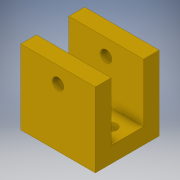
# Autodesk Inventor part: BracketForEndOfArm
Saved by Autodesk Inventor 2017 SP1 (Build 210196100, 196)
## iProperties
Created: 2016-06-07
Part Number: BracketForEndOfArm
Material: Generic
Document SubType Name: Modeling
Designer: steele
Density: 1 g/cm^3
Appearance: Gold
Author: steele
Autodesk Inventor part; units mm, degrees
ref_plane "YZ Plane" through (0, 0, 0) normal (1, 0, 0) x (0, 1, 0)
ref_plane "XZ Plane" through (0, 0, 0) normal (0, 1, 0) x (-1, 0, 0)
ref_plane "XY Plane" through (0, 0, 0) normal (0, 0, 1) x (1, 0, 0)
sketch "Sketch2" plane through (0, 0, 0) normal (1, 0, 0) x (0, 1, 0)
  line L0 (0, 0) -> (0, -19.05)
  line L1 (0, -19.05) -> (44.45, -19.05)
  line L2 (44.45, -19.05) -> (44.45, -9.652)
  line L3 (44.45, -9.652) -> (9.525, -9.652)
  line L4 (9.525, -9.652) -> (9.525, 0)
  line L5 (9.525, 0) -> (0, 0) construction
  line L6 (0, 0) -> (0, 19.05)
  line L7 (0, 19.05) -> (44.45, 19.05)
  line L8 (44.45, 19.05) -> (44.45, 9.652)
  line L9 (44.45, 9.652) -> (9.525, 9.652)
  line L10 (9.525, 9.652) -> (9.525, 0)
  dimension "d5" = 44.45
  dimension "d7" = 9.398
  dimension "d8" = 9.525
  dimension "d42" = 9.652
  constraints: 22 end point, 4 symmetric about line, 3 perpendicular, 2 vertical, 1 horizontal
  measures "d5" distance of L0.end L1.end
  measures "d7" distance between parallel lines of L1 L3
  measures "d8" distance between parallel lines of L0 L4
  measures "d42" distance from line of L0.start L3
extrude "Extrusion2" add sketch "Sketch2" along normal mid plane 44.45
sketch "Sketch3" plane through (-22.225, 0, 19.05) normal (0, 0, 1) x (1, 0, 0)
  line L0 (0, 44.45) -> (44.45, 44.45) projected
  line L1 (22.225, 44.45) -> (22.225, 0) construction
  point P0 (22.225, 34.925)
  dimension "d19" = 9.525
  constraints: 2 end point, 1 midpoint, 1 point on line, 1 vertical
  measures "d19" distance from line of point (22.225, 34.925) L0
hole "Hole2" at (0, 34.925, 19.05) direction (0, 0, -1) diameter 6.7564 end through all clearance for "Flat Head Machine Screw (82)" size "1/4" standard "Ansi Unified Screw Threads"
sketch "Sketch4" plane through (-22.225, 0, -19.05) normal (0, -1, 0) x (1, 0, 0)
  line L0 (44.45, 9.398) -> (44.45, 28.702) construction
  line L1 (44.45, 19.05) -> (0, 19.05) construction
  line L2 (0, 28.702) -> (0, 9.398) construction
  line L3 (44.45, 38.1) -> (44.45, 0) construction
  line L4 (19.05, 19.05) -> (-25.4, 19.05) construction
  point P0 (22.225, 19.05)
  point P1 (34.925, 19.05)
  point P2 (9.525, 19.05)
  dimension "d27" = 9.525
  dimension "d30" = 25.4
  constraints: 4 end point, 2 midpoint, 2 point on line, 1 collinear, 1 horizontal, 3 other
  measures "d27" distance from line of L3 point (34.925, 19.05)
  measures "d30" distance of point (34.925, 19.05) point (9.525, 19.05)
hole "Hole3" at (12.7, 0, 0) at (-12.7, 0, 0) direction (0, 1, 0) diameter 6.7564 end through all clearance for "Flat Head Machine Screw (82)" size "1/4" standard "Ansi Unified Screw Threads"
body "Solid2"
